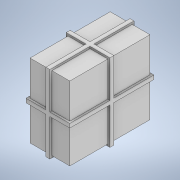
# Autodesk Inventor part: Motor
Saved by Autodesk Inventor 2022 (Build 260153000, 153)
## iProperties
Created: 2022-04-26
Part Number: Motor
Material: Generic
Document SubType Name: Modeling
Designer: dirks
Density: 1 g/cm^3
Appearance: Default
Author: dirks
Autodesk Inventor part; units mm, degrees
ref_plane "YZ Plane" through (0, 0, 0) normal (1, 0, 0) x (0, 1, 0)
ref_plane "XZ Plane" through (0, 0, 0) normal (0, 1, 0) x (-1, 0, 0)
ref_plane "XY Plane" through (0, 0, 0) normal (0, 0, 1) x (1, 0, 0)
sketch "Sketch1" plane through (0, 0, 0) normal (0, 1, 0) x (-1, 0, 0)
  line L0 (0, 0) -> (-20, 0)
  line L1 (-20, 0) -> (-20, -40.3)
  line L2 (-20, -40.3) -> (0, -40.3)
  line L3 (0, -40.3) -> (0, 0)
  dimension "d0" = 20
  dimension "d1" = 40.3
  constraints: 8 end point, 2 parallel, 1 horizontal, 1 perpendicular
  measures "d0" distance of L2.end L1.end
  measures "d1" distance of L1.end L0.end
extrude "Extrusion1" add sketch "Sketch1" along normal blind 37
sketch "Sketch2" plane through (20, 0, 0) normal (1, 0, 0) x (0, 0, -1)
  line L0 (0, 0) -> (40.3, 0) projected
  line L1 (40.3, 0) -> (40.3, 37) projected
  line L2 (21.15, 37) -> (19.15, 37)
  line L3 (19.15, 37) -> (19.15, 0)
  line L4 (19.15, 0) -> (21.15, 0)
  line L5 (21.15, 0) -> (21.15, 37)
  line L6 (0, 37) -> (40.3, 37) projected
  line L7 (0, 19.5) -> (40.3, 19.5)
  line L8 (40.3, 19.5) -> (40.3, 17.5)
  line L9 (40.3, 17.5) -> (0, 17.5)
  line L10 (0, 17.5) -> (0, 19.5)
  line L11 (0, 0) -> (0, 37) projected
  point P0 (19.15, 19.5)
  point P1 (19.15, 17.5)
  point P2 (21.15, 17.5)
  point P3 (21.15, 19.5)
  dimension "d5" = 2
  dimension "d6" = 19.15
  dimension "d7" = 0
  dimension "d9" = 2
  dimension "d10" = 17.5
  dimension "d11" = 0
  constraints: 16 end point, 4 parallel, 2 horizontal, 2 perpendicular, 2 point on line
  measures "d5" distance of L4.end L3.end
  measures "d6" distance between parallel lines of L1 L5
  measures "d7" distance between parallel lines of L6 L2
  measures "d9" distance of L7.end L8.end
  measures "d10" distance between parallel lines of L6 L7
  measures "d11" distance between parallel lines of L11 L10
extrude "Extrusion2" add sketch "Sketch2" along normal blind 1 contours L3 L9 L5 L0 | L10 L7 L3 L9 | L3 L7 L5 L9 | L5 L7 L1 L9 | L3 L2 L5 L7
sketch "Sketch3" plane through (0, 0, 0) normal (0, -1, 0) x (1, 0, 0)
  line L0 (0, 0) -> (20, 0) projected
  line L1 (0, -40.3) -> (0, 0) projected
  line L2 (20, -40.3) -> (0, -40.3) projected
  line L3 (20, -21.15) -> (21, -21.15) projected
  line L4 (21, -19.15) -> (21, -21.15) projected
  line L5 (20, -19.15) -> (21, -19.15) projected
  line L6 (21, -19.15) -> (0, -19.15)
  line L7 (0, -19.15) -> (0, -21.15)
  line L8 (0, -21.15) -> (21, -21.15)
  line L9 (21, -21.15) -> (21, -19.15)
  line L10 (0, 0) -> (20, 0) projected
  line L11 (11, 0) -> (9, 0)
  line L12 (9, 0) -> (9, -40.3)
  line L13 (9, -40.3) -> (11, -40.3)
  line L14 (11, -40.3) -> (11, 0)
  line L15 (9, -40.3) -> (9, 0)
  point P0 (9, -21.15)
  point P1 (11, -21.15)
  point P2 (11, -19.15)
  point P3 (9, -19.15)
  dimension "d14" = 10
  dimension "d15" = 12
  dimension "d16" = 0
  constraints: 18 end point, 5 equal length, 3 point on line, 2 horizontal, 2 perpendicular
  measures "d14" distance between parallel lines of L4 L14
  measures "d15" distance between parallel lines of L4 L12
  measures "d16" distance between parallel lines of L3 L8
extrude "Extrusion3" add sketch "Sketch3" along normal blind 1 contours L0 L14 L6 L12 | L6 L12 L8 L1 | L6 L14 L8 L12 | L6 L5 L4 L3 L8 L14 | L8 L14 L2 L12
sketch "Sketch4" plane through (20, 37, -40.3) normal (0, 0, -1) x (-1, 0, 0)
  line L0 (9, -37) -> (9, -38) projected
  line L1 (11, -38) -> (9, -38) projected
  line L2 (11, -37) -> (11, -38) projected
  line L3 (20, -37) -> (20, 0) projected
  line L4 (0, 0) -> (20, 0) projected
  line L5 (0, -17.5) -> (-1, -17.5) projected
  line L6 (-1, -19.5) -> (-1, -17.5) projected
  line L7 (0, -19.5) -> (-1, -19.5) projected
  line L8 (9, -38) -> (11, -38)
  line L9 (11, -38) -> (11, 0)
  line L10 (11, 0) -> (9, 0)
  line L11 (9, 0) -> (9, -38)
  line L12 (-1, -19.5) -> (20, -19.5)
  line L13 (20, -19.5) -> (20, -17.5)
  line L14 (20, -17.5) -> (-1, -17.5)
  line L15 (-1, -17.5) -> (-1, -19.5)
  point P0 (11, -17.5)
  point P1 (9, -17.5)
  point P2 (9, -19.5)
  point P3 (11, -19.5)
  constraints: 16 end point, 4 parallel, 2 horizontal, 2 perpendicular, 1 point on line
extrude "Extrusion4" add sketch "Sketch4" along normal blind 1 contours L11 L12 L9 L2 L1 L0 | L12 L7 L6 L5 L14 L11 | L11 L14 L9 L12 | L11 L4 L9 L14 | L9 L14 L3 L12
sketch "Sketch5" plane through (0, 37, 0) normal (0, 1, 0) x (1, 0, 0)
  line L0 (20, 19.15) -> (21, 19.15) projected
  line L1 (21, 21.15) -> (21, 19.15) projected
  line L2 (20, 21.15) -> (21, 21.15) projected
  line L3 (11, 40.3) -> (11, 41.3) projected
  line L4 (9, 41.3) -> (11, 41.3) projected
  line L5 (9, 40.3) -> (9, 41.3) projected
  line L6 (0, 40.3) -> (0, 0) projected
  line L7 (0, 0) -> (20, 0) projected
  line L8 (9, 0) -> (9, 19.15) projected
  line L9 (11, 41.3) -> (9, 41.3)
  line L10 (9, 41.3) -> (9, 0)
  line L11 (9, 0) -> (11, 0)
  line L12 (11, 0) -> (11, 41.3)
  line L13 (9, 19.15) -> (0, 19.15) projected
  line L14 (21, 21.15) -> (0, 21.15)
  line L15 (0, 21.15) -> (0, 19.15)
  line L16 (0, 19.15) -> (21, 19.15)
  line L17 (21, 19.15) -> (21, 21.15)
  point P0 (11, 19.15)
  point P1 (11, 21.15)
  point P2 (9, 21.15)
  constraints: 16 end point, 4 parallel, 2 horizontal, 2 perpendicular
extrude "Extrusion5" add sketch "Sketch5" along normal blind 1 contours L16 L12 L14 L2 L1 L0 | L16 L10 L14 L12 | L12 L7 L8 L16 | L14 L10 L5 L4 L3 L12 | L13 L6 L14 L10
sketch "Sketch6" plane through (0, 0, 0) normal (0, 0, 1) x (1, 0, 0)
  line L0 (9, 0) -> (9, -1) projected
  line L1 (11, -1) -> (9, -1) projected
  line L2 (11, 0) -> (11, -1) projected
  line L3 (20, 17.5) -> (21, 17.5) projected
  line L4 (21, 19.5) -> (21, 17.5) projected
  line L5 (20, 19.5) -> (21, 19.5) projected
  line L6 (11, 37) -> (11, 38) projected
  line L7 (9, 38) -> (11, 38) projected
  line L8 (9, 37) -> (9, 38) projected
  line L9 (0, 0) -> (0, 37) projected
  line L10 (11, 37) -> (11, 38) projected
  line L11 (0, -1) -> (9, -1) projected
  line L12 (11, 38) -> (9, 38)
  line L13 (9, 38) -> (9, -1)
  line L14 (9, -1) -> (11, -1)
  line L15 (11, -1) -> (11, 38)
  line L16 (21, 19.5) -> (21, 17.5) projected
  line L17 (0, 0) -> (0, 17.5) projected
  line L18 (21, 19.5) -> (0, 19.5)
  line L19 (0, 19.5) -> (0, 17.5)
  line L20 (0, 17.5) -> (21, 17.5)
  line L21 (21, 17.5) -> (21, 19.5)
  point P0 (11, 17.5)
  point P1 (11, 19.5)
  point P2 (9, 19.5)
  point P3 (9, 17.5)
  constraints: 16 end point, 4 parallel, 2 horizontal, 2 perpendicular
extrude "Extrusion6" add sketch "Sketch6" along normal blind 1
sketch "Sketch7" plane through (0, 0, -40.3) normal (-1, 0, 0) x (0, 0, 1)
  line L0 (19.15, 0) -> (19.15, -1) projected
  line L1 (21.15, -1) -> (19.15, -1) projected
  line L2 (21.15, 0) -> (21.15, -1) projected
  line L3 (40.3, 17.5) -> (41.3, 17.5) projected
  line L4 (41.3, 19.5) -> (41.3, 17.5) projected
  line L5 (40.3, 19.5) -> (41.3, 19.5) projected
  line L6 (21.15, 37) -> (21.15, 38) projected
  line L7 (19.15, 38) -> (21.15, 38) projected
  line L8 (19.15, 37) -> (19.15, 38) projected
  line L9 (0, 19.5) -> (-1, 19.5) projected
  line L10 (-1, 17.5) -> (-1, 19.5) projected
  line L11 (0, 17.5) -> (-1, 17.5) projected
  line L12 (19.15, -1) -> (21.15, -1) projected
  line L13 (21.15, -1) -> (19.15, -1)
  line L14 (19.15, -1) -> (19.15, 38)
  line L15 (19.15, 38) -> (21.15, 38)
  line L16 (21.15, 38) -> (21.15, -1)
  line L17 (41.3, 17.5) -> (-1, 17.5)
  line L18 (-1, 17.5) -> (-1, 19.5)
  line L19 (-1, 19.5) -> (41.3, 19.5)
  line L20 (41.3, 19.5) -> (41.3, 17.5)
  point P0 (21.15, 19.5)
  point P1 (19.15, 19.5)
  point P2 (19.15, 17.5)
  point P3 (21.15, 17.5)
  constraints: 16 end point, 4 parallel, 2 horizontal, 2 perpendicular
extrude "Extrusion7" add sketch "Sketch7" along normal blind 1
sketch "Sketch8" plane through (0, 0, 0) normal (0, -1, 0) x (1, 0, 0)
  circle A0 centre (10, -4) radius 2
  point P0 (0, 0)
  dimension "d27" = 4
  constraints: 1 centre point
  measures "d27" diameter of A0
extrude "Extrusion8" add sketch "Sketch8" along normal blind 2
body "Solid1"
